Autodesk Fusion 360 part; units mm, degrees
(part 3 of 6)
  arc A637 (41.675, 81.5) -> (38.5, 78.325) centre (41.675, 78.325) ccw
  arc A638 (57.5, 78.325) -> (54.325, 81.5) centre (54.325, 78.325) ccw
  line L961 (54.325, 62.5) -> (41.675, 62.5)
  line L962 (41.675, 81.5) -> (54.325, 81.5)
  arc A639 (38.5, 65.675) -> (41.675, 62.5) centre (41.675, 65.675) ccw
  line L963 (38.5, 81.5) -> (57.5, 62.5) construction
  arc A640 (78.325, 62.5) -> (81.5, 65.675) centre (78.325, 65.675) ccw
  line L964 (62.5, 65.675) -> (62.5, 78.325)
  line L965 (81.5, 78.325) -> (81.5, 65.675)
  line L966 (81.5, 81.5) -> (62.5, 62.5) construction
  arc A641 (65.675, 81.5) -> (62.5, 78.325) centre (65.675, 78.325) ccw
  arc A642 (81.5, 78.325) -> (78.325, 81.5) centre (78.325, 78.325) ccw
  line L967 (78.325, 62.5) -> (65.675, 62.5)
  line L968 (65.675, 81.5) -> (78.325, 81.5)
  arc A643 (62.5, 65.675) -> (65.675, 62.5) centre (65.675, 65.675) ccw
  line L969 (62.5, 81.5) -> (81.5, 62.5) construction
  arc A644 (102.325, 62.5) -> (105.5, 65.675) centre (102.325, 65.675) ccw
  line L970 (86.5, 65.675) -> (86.5, 78.325)
  line L971 (105.5, 78.325) -> (105.5, 65.675)
  line L972 (105.5, 81.5) -> (86.5, 62.5) construction
  arc A645 (89.675, 81.5) -> (86.5, 78.325) centre (89.675, 78.325) ccw
  arc A646 (105.5, 78.325) -> (102.325, 81.5) centre (102.325, 78.325) ccw
  line L973 (102.325, 62.5) -> (89.675, 62.5)
  line L974 (89.675, 81.5) -> (102.325, 81.5)
  arc A647 (86.5, 65.675) -> (89.675, 62.5) centre (89.675, 65.675) ccw
  line L975 (86.5, 81.5) -> (105.5, 62.5) construction
  arc A648 (126.325, 62.5) -> (129.5, 65.675) centre (126.325, 65.675) ccw
  line L976 (110.5, 65.675) -> (110.5, 78.325)
  line L977 (129.5, 78.325) -> (129.5, 65.675)
  line L978 (129.5, 81.5) -> (110.5, 62.5) construction
  arc A649 (113.675, 81.5) -> (110.5, 78.325) centre (113.675, 78.325) ccw
  arc A650 (129.5, 78.325) -> (126.325, 81.5) centre (126.325, 78.325) ccw
  line L979 (126.325, 62.5) -> (113.675, 62.5)
  line L980 (113.675, 81.5) -> (126.325, 81.5)
  arc A651 (110.5, 65.675) -> (113.675, 62.5) centre (113.675, 65.675) ccw
  line L981 (110.5, 81.5) -> (129.5, 62.5) construction
  arc A652 (150.325, 62.5) -> (153.5, 65.675) centre (150.325, 65.675) ccw
  line L982 (134.5, 65.675) -> (134.5, 78.325)
  line L983 (153.5, 78.325) -> (153.5, 65.675)
  line L984 (153.5, 81.5) -> (134.5, 62.5) construction
  arc A653 (137.675, 81.5) -> (134.5, 78.325) centre (137.675, 78.325) ccw
  arc A654 (153.5, 78.325) -> (150.325, 81.5) centre (150.325, 78.325) ccw
  line L985 (150.325, 62.5) -> (137.675, 62.5)
  line L986 (137.675, 81.5) -> (150.325, 81.5)
  arc A655 (134.5, 65.675) -> (137.675, 62.5) centre (137.675, 65.675) ccw
  line L987 (134.5, 81.5) -> (153.5, 62.5) construction
  arc A656 (174.325, 62.5) -> (177.5, 65.675) centre (174.325, 65.675) ccw
  line L988 (158.5, 65.675) -> (158.5, 78.325)
  line L989 (177.5, 78.325) -> (177.5, 65.675)
  line L990 (177.5, 81.5) -> (158.5, 62.5) construction
  arc A657 (161.675, 81.5) -> (158.5, 78.325) centre (161.675, 78.325) ccw
  arc A658 (177.5, 78.325) -> (174.325, 81.5) centre (174.325, 78.325) ccw
  line L991 (174.325, 62.5) -> (161.675, 62.5)
  line L992 (161.675, 81.5) -> (174.325, 81.5)
  arc A659 (158.5, 65.675) -> (161.675, 62.5) centre (161.675, 65.675) ccw
  line L993 (158.5, 81.5) -> (177.5, 62.5) construction
  arc A660 (-161.675, 86.5) -> (-158.5, 89.675) centre (-161.675, 89.675) ccw
  line L994 (-177.5, 89.675) -> (-177.5, 102.325)
  line L995 (-158.5, 102.325) -> (-158.5, 89.675)
  line L996 (-158.5, 105.5) -> (-177.5, 86.5) construction
  arc A661 (-174.325, 105.5) -> (-177.5, 102.325) centre (-174.325, 102.325) ccw
  arc A662 (-158.5, 102.325) -> (-161.675, 105.5) centre (-161.675, 102.325) ccw
  line L997 (-161.675, 86.5) -> (-174.325, 86.5)
  line L998 (-174.325, 105.5) -> (-161.675, 105.5)
  arc A663 (-177.5, 89.675) -> (-174.325, 86.5) centre (-174.325, 89.675) ccw
  line L999 (-177.5, 105.5) -> (-158.5, 86.5) construction
  arc A664 (-137.675, 86.5) -> (-134.5, 89.675) centre (-137.675, 89.675) ccw
  line L1000 (-153.5, 89.675) -> (-153.5, 102.325)
  line L1001 (-134.5, 102.325) -> (-134.5, 89.675)
  line L1002 (-134.5, 105.5) -> (-153.5, 86.5) construction
  arc A665 (-150.325, 105.5) -> (-153.5, 102.325) centre (-150.325, 102.325) ccw
  arc A666 (-134.5, 102.325) -> (-137.675, 105.5) centre (-137.675, 102.325) ccw
  line L1003 (-137.675, 86.5) -> (-150.325, 86.5)
  line L1004 (-150.325, 105.5) -> (-137.675, 105.5)
  arc A667 (-153.5, 89.675) -> (-150.325, 86.5) centre (-150.325, 89.675) ccw
  line L1005 (-153.5, 105.5) -> (-134.5, 86.5) construction
  arc A668 (-113.675, 86.5) -> (-110.5, 89.675) centre (-113.675, 89.675) ccw
  line L1006 (-129.5, 89.675) -> (-129.5, 102.325)
  line L1007 (-110.5, 102.325) -> (-110.5, 89.675)
  line L1008 (-110.5, 105.5) -> (-129.5, 86.5) construction
  arc A669 (-126.325, 105.5) -> (-129.5, 102.325) centre (-126.325, 102.325) ccw
  arc A670 (-110.5, 102.325) -> (-113.675, 105.5) centre (-113.675, 102.325) ccw
  line L1009 (-113.675, 86.5) -> (-126.325, 86.5)
  line L1010 (-126.325, 105.5) -> (-113.675, 105.5)
  arc A671 (-129.5, 89.675) -> (-126.325, 86.5) centre (-126.325, 89.675) ccw
  line L1011 (-129.5, 105.5) -> (-110.5, 86.5) construction
  arc A672 (-89.675, 86.5) -> (-86.5, 89.675) centre (-89.675, 89.675) ccw
  line L1012 (-105.5, 89.675) -> (-105.5, 102.325)
  line L1013 (-86.5, 102.325) -> (-86.5, 89.675)
  line L1014 (-86.5, 105.5) -> (-105.5, 86.5) construction
  arc A673 (-102.325, 105.5) -> (-105.5, 102.325) centre (-102.325, 102.325) ccw
  arc A674 (-86.5, 102.325) -> (-89.675, 105.5) centre (-89.675, 102.325) ccw
  line L1015 (-89.675, 86.5) -> (-102.325, 86.5)
  line L1016 (-102.325, 105.5) -> (-89.675, 105.5)
  arc A675 (-105.5, 89.675) -> (-102.325, 86.5) centre (-102.325, 89.675) ccw
  line L1017 (-105.5, 105.5) -> (-86.5, 86.5) construction
  arc A676 (-65.675, 86.5) -> (-62.5, 89.675) centre (-65.675, 89.675) ccw
  line L1018 (-81.5, 89.675) -> (-81.5, 102.325)
  line L1019 (-62.5, 102.325) -> (-62.5, 89.675)
  line L1020 (-62.5, 105.5) -> (-81.5, 86.5) construction
  arc A677 (-78.325, 105.5) -> (-81.5, 102.325) centre (-78.325, 102.325) ccw
  arc A678 (-62.5, 102.325) -> (-65.675, 105.5) centre (-65.675, 102.325) ccw
  line L1021 (-65.675, 86.5) -> (-78.325, 86.5)
  line L1022 (-78.325, 105.5) -> (-65.675, 105.5)
  arc A679 (-81.5, 89.675) -> (-78.325, 86.5) centre (-78.325, 89.675) ccw
  line L1023 (-81.5, 105.5) -> (-62.5, 86.5) construction
  arc A680 (-41.675, 86.5) -> (-38.5, 89.675) centre (-41.675, 89.675) ccw
  line L1024 (-57.5, 89.675) -> (-57.5, 102.325)
  line L1025 (-38.5, 102.325) -> (-38.5, 89.675)
  line L1026 (-38.5, 105.5) -> (-57.5, 86.5) construction
  arc A681 (-54.325, 105.5) -> (-57.5, 102.325) centre (-54.325, 102.325) ccw
  arc A682 (-38.5, 102.325) -> (-41.675, 105.5) centre (-41.675, 102.325) ccw
  line L1027 (-41.675, 86.5) -> (-54.325, 86.5)
  line L1028 (-54.325, 105.5) -> (-41.675, 105.5)
  arc A683 (-57.5, 89.675) -> (-54.325, 86.5) centre (-54.325, 89.675) ccw
  line L1029 (-57.5, 105.5) -> (-38.5, 86.5) construction
  arc A684 (-17.675, 86.5) -> (-14.5, 89.675) centre (-17.675, 89.675) ccw
  line L1030 (-33.5, 89.675) -> (-33.5, 102.325)
  line L1031 (-14.5, 102.325) -> (-14.5, 89.675)
  line L1032 (-14.5, 105.5) -> (-33.5, 86.5) construction
  arc A685 (-30.325, 105.5) -> (-33.5, 102.325) centre (-30.325, 102.325) ccw
  arc A686 (-14.5, 102.325) -> (-17.675, 105.5) centre (-17.675, 102.325) ccw
  line L1033 (-17.675, 86.5) -> (-30.325, 86.5)
  line L1034 (-30.325, 105.5) -> (-17.675, 105.5)
  arc A687 (-33.5, 89.675) -> (-30.325, 86.5) centre (-30.325, 89.675) ccw
  line L1035 (-33.5, 105.5) -> (-14.5, 86.5) construction
  arc A688 (6.325, 86.5) -> (9.5, 89.675) centre (6.325, 89.675) ccw
  line L1036 (-9.5, 89.675) -> (-9.5, 102.325)
  line L1037 (9.5, 102.325) -> (9.5, 89.675)
  line L1038 (9.5, 105.5) -> (-9.5, 86.5) construction
  arc A689 (-6.325, 105.5) -> (-9.5, 102.325) centre (-6.325, 102.325) ccw
  arc A690 (9.5, 102.325) -> (6.325, 105.5) centre (6.325, 102.325) ccw
  line L1039 (6.325, 86.5) -> (-6.325, 86.5)
  line L1040 (-6.325, 105.5) -> (6.325, 105.5)
  arc A691 (-9.5, 89.675) -> (-6.325, 86.5) centre (-6.325, 89.675) ccw
  line L1041 (-9.5, 105.5) -> (9.5, 86.5) construction
  arc A692 (30.325, 86.5) -> (33.5, 89.675) centre (30.325, 89.675) ccw
  line L1042 (14.5, 89.675) -> (14.5, 102.325)
  line L1043 (33.5, 102.325) -> (33.5, 89.675)
  line L1044 (33.5, 105.5) -> (14.5, 86.5) construction
  arc A693 (17.675, 105.5) -> (14.5, 102.325) centre (17.675, 102.325) ccw
  arc A694 (33.5, 102.325) -> (30.325, 105.5) centre (30.325, 102.325) ccw
  line L1045 (30.325, 86.5) -> (17.675, 86.5)
  line L1046 (17.675, 105.5) -> (30.325, 105.5)
  arc A695 (14.5, 89.675) -> (17.675, 86.5) centre (17.675, 89.675) ccw
  line L1047 (14.5, 105.5) -> (33.5, 86.5) construction
  arc A696 (54.325, 86.5) -> (57.5, 89.675) centre (54.325, 89.675) ccw
  line L1048 (38.5, 89.675) -> (38.5, 102.325)
  line L1049 (57.5, 102.325) -> (57.5, 89.675)
  line L1050 (57.5, 105.5) -> (38.5, 86.5) construction
  arc A697 (41.675, 105.5) -> (38.5, 102.325) centre (41.675, 102.325) ccw
  arc A698 (57.5, 102.325) -> (54.325, 105.5) centre (54.325, 102.325) ccw
  line L1051 (54.325, 86.5) -> (41.675, 86.5)
  line L1052 (41.675, 105.5) -> (54.325, 105.5)
  arc A699 (38.5, 89.675) -> (41.675, 86.5) centre (41.675, 89.675) ccw
  line L1053 (38.5, 105.5) -> (57.5, 86.5) construction
  arc A700 (78.325, 86.5) -> (81.5, 89.675) centre (78.325, 89.675) ccw
  line L1054 (62.5, 89.675) -> (62.5, 102.325)
  line L1055 (81.5, 102.325) -> (81.5, 89.675)
  line L1056 (81.5, 105.5) -> (62.5, 86.5) construction
  arc A701 (65.675, 105.5) -> (62.5, 102.325) centre (65.675, 102.325) ccw
  arc A702 (81.5, 102.325) -> (78.325, 105.5) centre (78.325, 102.325) ccw
  line L1057 (78.325, 86.5) -> (65.675, 86.5)
  line L1058 (65.675, 105.5) -> (78.325, 105.5)
  arc A703 (62.5, 89.675) -> (65.675, 86.5) centre (65.675, 89.675) ccw
  line L1059 (62.5, 105.5) -> (81.5, 86.5) construction
  arc A704 (102.325, 86.5) -> (105.5, 89.675) centre (102.325, 89.675) ccw
  line L1060 (86.5, 89.675) -> (86.5, 102.325)
  line L1061 (105.5, 102.325) -> (105.5, 89.675)
  line L1062 (105.5, 105.5) -> (86.5, 86.5) construction
  arc A705 (89.675, 105.5) -> (86.5, 102.325) centre (89.675, 102.325) ccw
  arc A706 (105.5, 102.325) -> (102.325, 105.5) centre (102.325, 102.325) ccw
  line L1063 (102.325, 86.5) -> (89.675, 86.5)
  line L1064 (89.675, 105.5) -> (102.325, 105.5)
  arc A707 (86.5, 89.675) -> (89.675, 86.5) centre (89.675, 89.675) ccw
  line L1065 (86.5, 105.5) -> (105.5, 86.5) construction
  arc A708 (126.325, 86.5) -> (129.5, 89.675) centre (126.325, 89.675) ccw
  line L1066 (110.5, 89.675) -> (110.5, 102.325)
  line L1067 (129.5, 102.325) -> (129.5, 89.675)
  line L1068 (129.5, 105.5) -> (110.5, 86.5) construction
  arc A709 (113.675, 105.5) -> (110.5, 102.325) centre (113.675, 102.325) ccw
  arc A710 (129.5, 102.325) -> (126.325, 105.5) centre (126.325, 102.325) ccw
  line L1069 (126.325, 86.5) -> (113.675, 86.5)
  line L1070 (113.675, 105.5) -> (126.325, 105.5)
  arc A711 (110.5, 89.675) -> (113.675, 86.5) centre (113.675, 89.675) ccw
  line L1071 (110.5, 105.5) -> (129.5, 86.5) construction
  arc A712 (150.325, 86.5) -> (153.5, 89.675) centre (150.325, 89.675) ccw
  line L1072 (134.5, 89.675) -> (134.5, 102.325)
  line L1073 (153.5, 102.325) -> (153.5, 89.675)
  line L1074 (153.5, 105.5) -> (134.5, 86.5) construction
  arc A713 (137.675, 105.5) -> (134.5, 102.325) centre (137.675, 102.325) ccw
  arc A714 (153.5, 102.325) -> (150.325, 105.5) centre (150.325, 102.325) ccw
  line L1075 (150.325, 86.5) -> (137.675, 86.5)
  line L1076 (137.675, 105.5) -> (150.325, 105.5)
  arc A715 (134.5, 89.675) -> (137.675, 86.5) centre (137.675, 89.675) ccw
  line L1077 (134.5, 105.5) -> (153.5, 86.5) construction
  arc A716 (174.325, 86.5) -> (177.5, 89.675) centre (174.325, 89.675) ccw
  line L1078 (158.5, 89.675) -> (158.5, 102.325)
  line L1079 (177.5, 102.325) -> (177.5, 89.675)
  line L1080 (177.5, 105.5) -> (158.5, 86.5) construction
  arc A717 (161.675, 105.5) -> (158.5, 102.325) centre (161.675, 102.325) ccw
  arc A718 (177.5, 102.325) -> (174.325, 105.5) centre (174.325, 102.325) ccw
  line L1081 (174.325, 86.5) -> (161.675, 86.5)
  line L1082 (161.675, 105.5) -> (174.325, 105.5)
  arc A719 (158.5, 89.675) -> (161.675, 86.5) centre (161.675, 89.675) ccw
  line L1083 (158.5, 105.5) -> (177.5, 86.5) construction
  arc A720 (-161.675, 110.5) -> (-158.5, 113.675) centre (-161.675, 113.675) ccw
  line L1084 (-177.5, 113.675) -> (-177.5, 126.325)
  line L1085 (-158.5, 126.325) -> (-158.5, 113.675)
  line L1086 (-158.5, 129.5) -> (-177.5, 110.5) construction
  arc A721 (-174.325, 129.5) -> (-177.5, 126.325) centre (-174.325, 126.325) ccw
  arc A722 (-158.5, 126.325) -> (-161.675, 129.5) centre (-161.675, 126.325) ccw
  line L1087 (-161.675, 110.5) -> (-174.325, 110.5)
  line L1088 (-174.325, 129.5) -> (-161.675, 129.5)
  arc A723 (-177.5, 113.675) -> (-174.325, 110.5) centre (-174.325, 113.675) ccw
  line L1089 (-177.5, 129.5) -> (-158.5, 110.5) construction
  arc A724 (-137.675, 110.5) -> (-134.5, 113.675) centre (-137.675, 113.675) ccw
  line L1090 (-153.5, 113.675) -> (-153.5, 126.325)
  line L1091 (-134.5, 126.325) -> (-134.5, 113.675)
  line L1092 (-134.5, 129.5) -> (-153.5, 110.5) construction
  arc A725 (-150.325, 129.5) -> (-153.5, 126.325) centre (-150.325, 126.325) ccw
  arc A726 (-134.5, 126.325) -> (-137.675, 129.5) centre (-137.675, 126.325) ccw
  line L1093 (-137.675, 110.5) -> (-150.325, 110.5)
  line L1094 (-150.325, 129.5) -> (-137.675, 129.5)
  arc A727 (-153.5, 113.675) -> (-150.325, 110.5) centre (-150.325, 113.675) ccw
  line L1095 (-153.5, 129.5) -> (-134.5, 110.5) construction
  arc A728 (-113.675, 110.5) -> (-110.5, 113.675) centre (-113.675, 113.675) ccw
  line L1096 (-129.5, 113.675) -> (-129.5, 126.325)
  line L1097 (-110.5, 126.325) -> (-110.5, 113.675)
  line L1098 (-110.5, 129.5) -> (-129.5, 110.5) construction
  arc A729 (-126.325, 129.5) -> (-129.5, 126.325) centre (-126.325, 126.325) ccw
  arc A730 (-110.5, 126.325) -> (-113.675, 129.5) centre (-113.675, 126.325) ccw
  line L1099 (-113.675, 110.5) -> (-126.325, 110.5)
  line L1100 (-126.325, 129.5) -> (-113.675, 129.5)
  arc A731 (-129.5, 113.675) -> (-126.325, 110.5) centre (-126.325, 113.675) ccw
  line L1101 (-129.5, 129.5) -> (-110.5, 110.5) construction
  arc A732 (-89.675, 110.5) -> (-86.5, 113.675) centre (-89.675, 113.675) ccw
  line L1102 (-105.5, 113.675) -> (-105.5, 126.325)
  line L1103 (-86.5, 126.325) -> (-86.5, 113.675)
  line L1104 (-86.5, 129.5) -> (-105.5, 110.5) construction
  arc A733 (-102.325, 129.5) -> (-105.5, 126.325) centre (-102.325, 126.325) ccw
  arc A734 (-86.5, 126.325) -> (-89.675, 129.5) centre (-89.675, 126.325) ccw
  line L1105 (-89.675, 110.5) -> (-102.325, 110.5)
  line L1106 (-102.325, 129.5) -> (-89.675, 129.5)
  arc A735 (-105.5, 113.675) -> (-102.325, 110.5) centre (-102.325, 113.675) ccw
  line L1107 (-105.5, 129.5) -> (-86.5, 110.5) construction
  arc A736 (-65.675, 110.5) -> (-62.5, 113.675) centre (-65.675, 113.675) ccw
  line L1108 (-81.5, 113.675) -> (-81.5, 126.325)
  line L1109 (-62.5, 126.325) -> (-62.5, 113.675)
  line L1110 (-62.5, 129.5) -> (-81.5, 110.5) construction
  arc A737 (-78.325, 129.5) -> (-81.5, 126.325) centre (-78.325, 126.325) ccw
  arc A738 (-62.5, 126.325) -> (-65.675, 129.5) centre (-65.675, 126.325) ccw
  line L1111 (-65.675, 110.5) -> (-78.325, 110.5)
  line L1112 (-78.325, 129.5) -> (-65.675, 129.5)
  arc A739 (-81.5, 113.675) -> (-78.325, 110.5) centre (-78.325, 113.675) ccw
  line L1113 (-81.5, 129.5) -> (-62.5, 110.5) construction
  arc A740 (-41.675, 110.5) -> (-38.5, 113.675) centre (-41.675, 113.675) ccw
  line L1114 (-57.5, 113.675) -> (-57.5, 126.325)
  line L1115 (-38.5, 126.325) -> (-38.5, 113.675)
  line L1116 (-38.5, 129.5) -> (-57.5, 110.5) construction
  arc A741 (-54.325, 129.5) -> (-57.5, 126.325) centre (-54.325, 126.325) ccw
  arc A742 (-38.5, 126.325) -> (-41.675, 129.5) centre (-41.675, 126.325) ccw
  line L1117 (-41.675, 110.5) -> (-54.325, 110.5)
  line L1118 (-54.325, 129.5) -> (-41.675, 129.5)
  arc A743 (-57.5, 113.675) -> (-54.325, 110.5) centre (-54.325, 113.675) ccw
  line L1119 (-57.5, 129.5) -> (-38.5, 110.5) construction
  arc A744 (-17.675, 110.5) -> (-14.5, 113.675) centre (-17.675, 113.675) ccw
  line L1120 (-33.5, 113.675) -> (-33.5, 126.325)
  line L1121 (-14.5, 126.325) -> (-14.5, 113.675)
  line L1122 (-14.5, 129.5) -> (-33.5, 110.5) construction
  arc A745 (-30.325, 129.5) -> (-33.5, 126.325) centre (-30.325, 126.325) ccw
  arc A746 (-14.5, 126.325) -> (-17.675, 129.5) centre (-17.675, 126.325) ccw
  line L1123 (-17.675, 110.5) -> (-30.325, 110.5)
  line L1124 (-30.325, 129.5) -> (-17.675, 129.5)
  arc A747 (-33.5, 113.675) -> (-30.325, 110.5) centre (-30.325, 113.675) ccw
  line L1125 (-33.5, 129.5) -> (-14.5, 110.5) construction
  arc A748 (6.325, 110.5) -> (9.5, 113.675) centre (6.325, 113.675) ccw
  line L1126 (-9.5, 113.675) -> (-9.5, 126.325)
  line L1127 (9.5, 126.325) -> (9.5, 113.675)
  line L1128 (9.5, 129.5) -> (-9.5, 110.5) construction
  arc A749 (-6.325, 129.5) -> (-9.5, 126.325) centre (-6.325, 126.325) ccw
  arc A750 (9.5, 126.325) -> (6.325, 129.5) centre (6.325, 126.325) ccw
  line L1129 (6.325, 110.5) -> (-6.325, 110.5)
  line L1130 (-6.325, 129.5) -> (6.325, 129.5)
  arc A751 (-9.5, 113.675) -> (-6.325, 110.5) centre (-6.325, 113.675) ccw
  line L1131 (-9.5, 129.5) -> (9.5, 110.5) construction
  arc A752 (30.325, 110.5) -> (33.5, 113.675) centre (30.325, 113.675) ccw
  line L1132 (14.5, 113.675) -> (14.5, 126.325)
  line L1133 (33.5, 126.325) -> (33.5, 113.675)
  line L1134 (33.5, 129.5) -> (14.5, 110.5) construction
  arc A753 (17.675, 129.5) -> (14.5, 126.325) centre (17.675, 126.325) ccw
  arc A754 (33.5, 126.325) -> (30.325, 129.5) centre (30.325, 126.325) ccw
  line L1135 (30.325, 110.5) -> (17.675, 110.5)
  line L1136 (17.675, 129.5) -> (30.325, 129.5)
  arc A755 (14.5, 113.675) -> (17.675, 110.5) centre (17.675, 113.675) ccw
  line L1137 (14.5, 129.5) -> (33.5, 110.5) construction
  arc A756 (54.325, 110.5) -> (57.5, 113.675) centre (54.325, 113.675) ccw
  line L1138 (38.5, 113.675) -> (38.5, 126.325)
  line L1139 (57.5, 126.325) -> (57.5, 113.675)
  line L1140 (57.5, 129.5) -> (38.5, 110.5) construction
  arc A757 (41.675, 129.5) -> (38.5, 126.325) centre (41.675, 126.325) ccw
  arc A758 (57.5, 126.325) -> (54.325, 129.5) centre (54.325, 126.325) ccw
  line L1141 (54.325, 110.5) -> (41.675, 110.5)
  line L1142 (41.675, 129.5) -> (54.325, 129.5)
  arc A759 (38.5, 113.675) -> (41.675, 110.5) centre (41.675, 113.675) ccw
  line L1143 (38.5, 129.5) -> (57.5, 110.5) construction
  arc A760 (78.325, 110.5) -> (81.5, 113.675) centre (78.325, 113.675) ccw
  line L1144 (62.5, 113.675) -> (62.5, 126.325)
  line L1145 (81.5, 126.325) -> (81.5, 113.675)
  line L1146 (81.5, 129.5) -> (62.5, 110.5) construction
  arc A761 (65.675, 129.5) -> (62.5, 126.325) centre (65.675, 126.325) ccw
  arc A762 (81.5, 126.325) -> (78.325, 129.5) centre (78.325, 126.325) ccw
  line L1147 (78.325, 110.5) -> (65.675, 110.5)
  line L1148 (65.675, 129.5) -> (78.325, 129.5)
  arc A763 (62.5, 113.675) -> (65.675, 110.5) centre (65.675, 113.675) ccw
  line L1149 (62.5, 129.5) -> (81.5, 110.5) construction
  arc A764 (102.325, 110.5) -> (105.5, 113.675) centre (102.325, 113.675) ccw
  line L1150 (86.5, 113.675) -> (86.5, 126.325)
  line L1151 (105.5, 126.325) -> (105.5, 113.675)
  line L1152 (105.5, 129.5) -> (86.5, 110.5) construction
  arc A765 (89.675, 129.5) -> (86.5, 126.325) centre (89.675, 126.325) ccw
  arc A766 (105.5, 126.325) -> (102.325, 129.5) centre (102.325, 126.325) ccw
  line L1153 (102.325, 110.5) -> (89.675, 110.5)
  line L1154 (89.675, 129.5) -> (102.325, 129.5)
  arc A767 (86.5, 113.675) -> (89.675, 110.5) centre (89.675, 113.675) ccw
  line L1155 (86.5, 129.5) -> (105.5, 110.5) construction
  arc A768 (126.325, 110.5) -> (129.5, 113.675) centre (126.325, 113.675) ccw
  line L1156 (110.5, 113.675) -> (110.5, 126.325)
  line L1157 (129.5, 126.325) -> (129.5, 113.675)
  line L1158 (129.5, 129.5) -> (110.5, 110.5) construction
  arc A769 (113.675, 129.5) -> (110.5, 126.325) centre (113.675, 126.325) ccw
  arc A770 (129.5, 126.325) -> (126.325, 129.5) centre (126.325, 126.325) ccw
  line L1159 (126.325, 110.5) -> (113.675, 110.5)
  line L1160 (113.675, 129.5) -> (126.325, 129.5)
  arc A771 (110.5, 113.675) -> (113.675, 110.5) centre (113.675, 113.675) ccw
  line L1161 (110.5, 129.5) -> (129.5, 110.5) construction
  arc A772 (150.325, 110.5) -> (153.5, 113.675) centre (150.325, 113.675) ccw
  line L1162 (134.5, 113.675) -> (134.5, 126.325)
  line L1163 (153.5, 126.325) -> (153.5, 113.675)
  line L1164 (153.5, 129.5) -> (134.5, 110.5) construction
  arc A773 (137.675, 129.5) -> (134.5, 126.325) centre (137.675, 126.325) ccw
  arc A774 (153.5, 126.325) -> (150.325, 129.5) centre (150.325, 126.325) ccw
  line L1165 (150.325, 110.5) -> (137.675, 110.5)
  line L1166 (137.675, 129.5) -> (150.325, 129.5)
  arc A775 (134.5, 113.675) -> (137.675, 110.5) centre (137.675, 113.675) ccw
  line L1167 (134.5, 129.5) -> (153.5, 110.5) construction
  arc A776 (174.325, 110.5) -> (177.5, 113.675) centre (174.325, 113.675) ccw
  line L1168 (158.5, 113.675) -> (158.5, 126.325)
  line L1169 (177.5, 126.325) -> (177.5, 113.675)
  line L1170 (177.5, 129.5) -> (158.5, 110.5) construction
  arc A777 (161.675, 129.5) -> (158.5, 126.325) centre (161.675, 126.325) ccw
  arc A778 (177.5, 126.325) -> (174.325, 129.5) centre (174.325, 126.325) ccw
  line L1171 (174.325, 110.5) -> (161.675, 110.5)
  line L1172 (161.675, 129.5) -> (174.325, 129.5)
  arc A779 (158.5, 113.675) -> (161.675, 110.5) centre (161.675, 113.675) ccw
  line L1173 (158.5, 129.5) -> (177.5, 110.5) construction
  arc A780 (-161.675, 134.5) -> (-158.5, 137.675) centre (-161.675, 137.675) ccw
  line L1174 (-177.5, 137.675) -> (-177.5, 150.325)
  line L1175 (-158.5, 150.325) -> (-158.5, 137.675)
  line L1176 (-158.5, 153.5) -> (-177.5, 134.5) construction
  arc A781 (-174.325, 153.5) -> (-177.5, 150.325) centre (-174.325, 150.325) ccw
  arc A782 (-158.5, 150.325) -> (-161.675, 153.5) centre (-161.675, 150.325) ccw
  line L1177 (-161.675, 134.5) -> (-174.325, 134.5)
  line L1178 (-174.325, 153.5) -> (-161.675, 153.5)
  arc A783 (-177.5, 137.675) -> (-174.325, 134.5) centre (-174.325, 137.675) ccw
  line L1179 (-177.5, 153.5) -> (-158.5, 134.5) construction
  arc A784 (-137.675, 134.5) -> (-134.5, 137.675) centre (-137.675, 137.675) ccw
  line L1180 (-153.5, 137.675) -> (-153.5, 150.325)
  line L1181 (-134.5, 150.325) -> (-134.5, 137.675)
  line L1182 (-134.5, 153.5) -> (-153.5, 134.5) construction
  arc A785 (-150.325, 153.5) -> (-153.5, 150.325) centre (-150.325, 150.325) ccw
  arc A786 (-134.5, 150.325) -> (-137.675, 153.5) centre (-137.675, 150.325) ccw
  line L1183 (-137.675, 134.5) -> (-150.325, 134.5)
  line L1184 (-150.325, 153.5) -> (-137.675, 153.5)
  arc A787 (-153.5, 137.675) -> (-150.325, 134.5) centre (-150.325, 137.675) ccw
  line L1185 (-153.5, 153.5) -> (-134.5, 134.5) construction
  arc A788 (-113.675, 134.5) -> (-110.5, 137.675) centre (-113.675, 137.675) ccw
  line L1186 (-129.5, 137.675) -> (-129.5, 150.325)
  line L1187 (-110.5, 150.325) -> (-110.5, 137.675)
  line L1188 (-110.5, 153.5) -> (-129.5, 134.5) construction
  arc A789 (-126.325, 153.5) -> (-129.5, 150.325) centre (-126.325, 150.325) ccw
  arc A790 (-110.5, 150.325) -> (-113.675, 153.5) centre (-113.675, 150.325) ccw
  line L1189 (-113.675, 134.5) -> (-126.325, 134.5)
  line L1190 (-126.325, 153.5) -> (-113.675, 153.5)
  arc A791 (-129.5, 137.675) -> (-126.325, 134.5) centre (-126.325, 137.675) ccw
  line L1191 (-129.5, 153.5) -> (-110.5, 134.5) construction
  arc A792 (-89.675, 134.5) -> (-86.5, 137.675) centre (-89.675, 137.675) ccw
  line L1192 (-105.5, 137.675) -> (-105.5, 150.325)
  line L1193 (-86.5, 150.325) -> (-86.5, 137.675)
  line L1194 (-86.5, 153.5) -> (-105.5, 134.5) construction
  arc A793 (-102.325, 153.5) -> (-105.5, 150.325) centre (-102.325, 150.325) ccw
  arc A794 (-86.5, 150.325) -> (-89.675, 153.5) centre (-89.675, 150.325) ccw
  line L1195 (-89.675, 134.5) -> (-102.325, 134.5)
  line L1196 (-102.325, 153.5) -> (-89.675, 153.5)
  arc A795 (-105.5, 137.675) -> (-102.325, 134.5) centre (-102.325, 137.675) ccw
  line L1197 (-105.5, 153.5) -> (-86.5, 134.5) construction
  arc A796 (-65.675, 134.5) -> (-62.5, 137.675) centre (-65.675, 137.675) ccw
  line L1198 (-81.5, 137.675) -> (-81.5, 150.325)
  line L1199 (-62.5, 150.325) -> (-62.5, 137.675)
  line L1200 (-62.5, 153.5) -> (-81.5, 134.5) construction
  arc A797 (-78.325, 153.5) -> (-81.5, 150.325) centre (-78.325, 150.325) ccw
  arc A798 (-62.5, 150.325) -> (-65.675, 153.5) centre (-65.675, 150.325) ccw
  line L1201 (-65.675, 134.5) -> (-78.325, 134.5)
  line L1202 (-78.325, 153.5) -> (-65.675, 153.5)
  arc A799 (-81.5, 137.675) -> (-78.325, 134.5) centre (-78.325, 137.675) ccw
  line L1203 (-81.5, 153.5) -> (-62.5, 134.5) construction
  arc A800 (-41.675, 134.5) -> (-38.5, 137.675) centre (-41.675, 137.675) ccw
  line L1204 (-57.5, 137.675) -> (-57.5, 150.325)
  line L1205 (-38.5, 150.325) -> (-38.5, 137.675)
  line L1206 (-38.5, 153.5) -> (-57.5, 134.5) construction
  arc A801 (-54.325, 153.5) -> (-57.5, 150.325) centre (-54.325, 150.325) ccw
  arc A802 (-38.5, 150.325) -> (-41.675, 153.5) centre (-41.675, 150.325) ccw
  line L1207 (-41.675, 134.5) -> (-54.325, 134.5)
  line L1208 (-54.325, 153.5) -> (-41.675, 153.5)
  arc A803 (-57.5, 137.675) -> (-54.325, 134.5) centre (-54.325, 137.675) ccw
  line L1209 (-57.5, 153.5) -> (-38.5, 134.5) construction
  arc A804 (-17.675, 134.5) -> (-14.5, 137.675) centre (-17.675, 137.675) ccw
  line L1210 (-33.5, 137.675) -> (-33.5, 150.325)
  line L1211 (-14.5, 150.325) -> (-14.5, 137.675)
  line L1212 (-14.5, 153.5) -> (-33.5, 134.5) construction
  arc A805 (-30.325, 153.5) -> (-33.5, 150.325) centre (-30.325, 150.325) ccw
  arc A806 (-14.5, 150.325) -> (-17.675, 153.5) centre (-17.675, 150.325) ccw
  line L1213 (-17.675, 134.5) -> (-30.325, 134.5)
  line L1214 (-30.325, 153.5) -> (-17.675, 153.5)
  arc A807 (-33.5, 137.675) -> (-30.325, 134.5) centre (-30.325, 137.675) ccw
  line L1215 (-33.5, 153.5) -> (-14.5, 134.5) construction
  arc A808 (6.325, 134.5) -> (9.5, 137.675) centre (6.325, 137.675) ccw
  line L1216 (-9.5, 137.675) -> (-9.5, 150.325)
  line L1217 (9.5, 150.325) -> (9.5, 137.675)
  line L1218 (9.5, 153.5) -> (-9.5, 134.5) construction
  arc A809 (-6.325, 153.5) -> (-9.5, 150.325) centre (-6.325, 150.325) ccw
  arc A810 (9.5, 150.325) -> (6.325, 153.5) centre (6.325, 150.325) ccw
  line L1219 (6.325, 134.5) -> (-6.325, 134.5)
  line L1220 (-6.325, 153.5) -> (6.325, 153.5)
  arc A811 (-9.5, 137.675) -> (-6.325, 134.5) centre (-6.325, 137.675) ccw
  line L1221 (-9.5, 153.5) -> (9.5, 134.5) construction
  arc A812 (30.325, 134.5) -> (33.5, 137.675) centre (30.325, 137.675) ccw
  line L1222 (14.5, 137.675) -> (14.5, 150.325)
  line L1223 (33.5, 150.325) -> (33.5, 137.675)
  line L1224 (33.5, 153.5) -> (14.5, 134.5) construction
  arc A813 (17.675, 153.5) -> (14.5, 150.325) centre (17.675, 150.325) ccw
  arc A814 (33.5, 150.325) -> (30.325, 153.5) centre (30.325, 150.325) ccw
  line L1225 (30.325, 134.5) -> (17.675, 134.5)
  line L1226 (17.675, 153.5) -> (30.325, 153.5)
  arc A815 (14.5, 137.675) -> (17.675, 134.5) centre (17.675, 137.675) ccw
  line L1227 (14.5, 153.5) -> (33.5, 134.5) construction
  arc A816 (54.325, 134.5) -> (57.5, 137.675) centre (54.325, 137.675) ccw
  line L1228 (38.5, 137.675) -> (38.5, 150.325)
  line L1229 (57.5, 150.325) -> (57.5, 137.675)
  line L1230 (57.5, 153.5) -> (38.5, 134.5) construction
  arc A817 (41.675, 153.5) -> (38.5, 150.325) centre (41.675, 150.325) ccw
  arc A818 (57.5, 150.325) -> (54.325, 153.5) centre (54.325, 150.325) ccw
  line L1231 (54.325, 134.5) -> (41.675, 134.5)
  line L1232 (41.675, 153.5) -> (54.325, 153.5)
  arc A819 (38.5, 137.675) -> (41.675, 134.5) centre (41.675, 137.675) ccw
  line L1233 (38.5, 153.5) -> (57.5, 134.5) construction
  arc A820 (78.325, 134.5) -> (81.5, 137.675) centre (78.325, 137.675) ccw
  line L1234 (62.5, 137.675) -> (62.5, 150.325)
  line L1235 (81.5, 150.325) -> (81.5, 137.675)
  line L1236 (81.5, 153.5) -> (62.5, 134.5) construction
  arc A821 (65.675, 153.5) -> (62.5, 150.325) centre (65.675, 150.325) ccw
  arc A822 (81.5, 150.325) -> (78.325, 153.5) centre (78.325, 150.325) ccw
  line L1237 (78.325, 134.5) -> (65.675, 134.5)
  line L1238 (65.675, 153.5) -> (78.325, 153.5)
  arc A823 (62.5, 137.675) -> (65.675, 134.5) centre (65.675, 137.675) ccw
  line L1239 (62.5, 153.5) -> (81.5, 134.5) construction
  arc A824 (102.325, 134.5) -> (105.5, 137.675) centre (102.325, 137.675) ccw
  line L1240 (86.5, 137.675) -> (86.5, 150.325)
  line L1241 (105.5, 150.325) -> (105.5, 137.675)
  line L1242 (105.5, 153.5) -> (86.5, 134.5) construction
  arc A825 (89.675, 153.5) -> (86.5, 150.325) centre (89.675, 150.325) ccw
  arc A826 (105.5, 150.325) -> (102.325, 153.5) centre (102.325, 150.325) ccw
  line L1243 (102.325, 134.5) -> (89.675, 134.5)
  line L1244 (89.675, 153.5) -> (102.325, 153.5)
  arc A827 (86.5, 137.675) -> (89.675, 134.5) centre (89.675, 137.675) ccw
  line L1245 (86.5, 153.5) -> (105.5, 134.5) construction
  arc A828 (126.325, 134.5) -> (129.5, 137.675) centre (126.325, 137.675) ccw
  line L1246 (110.5, 137.675) -> (110.5, 150.325)
  line L1247 (129.5, 150.325) -> (129.5, 137.675)
  line L1248 (129.5, 153.5) -> (110.5, 134.5) construction
  arc A829 (113.675, 153.5) -> (110.5, 150.325) centre (113.675, 150.325) ccw
  arc A830 (129.5, 150.325) -> (126.325, 153.5) centre (126.325, 150.325) ccw
  line L1249 (126.325, 134.5) -> (113.675, 134.5)
  line L1250 (113.675, 153.5) -> (126.325, 153.5)
  arc A831 (110.5, 137.675) -> (113.675, 134.5) centre (113.675, 137.675) ccw
  line L1251 (110.5, 153.5) -> (129.5, 134.5) construction
  arc A832 (150.325, 134.5) -> (153.5, 137.675) centre (150.325, 137.675) ccw
  line L1252 (134.5, 137.675) -> (134.5, 150.325)
  line L1253 (153.5, 150.325) -> (153.5, 137.675)
  line L1254 (153.5, 153.5) -> (134.5, 134.5) construction
  arc A833 (137.675, 153.5) -> (134.5, 150.325) centre (137.675, 150.325) ccw
  arc A834 (153.5, 150.325) -> (150.325, 153.5) centre (150.325, 150.325) ccw
  line L1255 (150.325, 134.5) -> (137.675, 134.5)
  line L1256 (137.675, 153.5) -> (150.325, 153.5)
  arc A835 (134.5, 137.675) -> (137.675, 134.5) centre (137.675, 137.675) ccw
  line L1257 (134.5, 153.5) -> (153.5, 134.5) construction
  arc A836 (174.325, 134.5) -> (177.5, 137.675) centre (174.325, 137.675) ccw
  line L1258 (158.5, 137.675) -> (158.5, 150.325)
  line L1259 (177.5, 150.325) -> (177.5, 137.675)
  line L1260 (177.5, 153.5) -> (158.5, 134.5) construction
  arc A837 (161.675, 153.5) -> (158.5, 150.325) centre (161.675, 150.325) ccw
  arc A838 (177.5, 150.325) -> (174.325, 153.5) centre (174.325, 150.325) ccw
  line L1261 (174.325, 134.5) -> (161.675, 134.5)
  line L1262 (161.675, 153.5) -> (174.325, 153.5)
  arc A839 (158.5, 137.675) -> (161.675, 134.5) centre (161.675, 137.675) ccw
  line L1263 (158.5, 153.5) -> (177.5, 134.5) construction
  arc A840 (-161.675, 158.5) -> (-158.5, 161.675) centre (-161.675, 161.675) ccw
  line L1264 (-177.5, 161.675) -> (-177.5, 174.325)
  line L1265 (-158.5, 174.325) -> (-158.5, 161.675)
  line L1266 (-158.5, 177.5) -> (-177.5, 158.5) construction
  arc A841 (-174.325, 177.5) -> (-177.5, 174.325) centre (-174.325, 174.325) ccw
  arc A842 (-158.5, 174.325) -> (-161.675, 177.5) centre (-161.675, 174.325) ccw
  line L1267 (-161.675, 158.5) -> (-174.325, 158.5)
  line L1268 (-174.325, 177.5) -> (-161.675, 177.5)
  arc A843 (-177.5, 161.675) -> (-174.325, 158.5) centre (-174.325, 161.675) ccw
  line L1269 (-177.5, 177.5) -> (-158.5, 158.5) construction
  arc A844 (-137.675, 158.5) -> (-134.5, 161.675) centre (-137.675, 161.675) ccw
  line L1270 (-153.5, 161.675) -> (-153.5, 174.325)
  line L1271 (-134.5, 174.325) -> (-134.5, 161.675)
  line L1272 (-134.5, 177.5) -> (-153.5, 158.5) construction
  arc A845 (-150.325, 177.5) -> (-153.5, 174.325) centre (-150.325, 174.325) ccw
  arc A846 (-134.5, 174.325) -> (-137.675, 177.5) centre (-137.675, 174.325) ccw
  line L1273 (-137.675, 158.5) -> (-150.325, 158.5)
  line L1274 (-150.325, 177.5) -> (-137.675, 177.5)
  arc A847 (-153.5, 161.675) -> (-150.325, 158.5) centre (-150.325, 161.675) ccw
  line L1275 (-153.5, 177.5) -> (-134.5, 158.5) construction
  arc A848 (-113.675, 158.5) -> (-110.5, 161.675) centre (-113.675, 161.675) ccw
  line L1276 (-129.5, 161.675) -> (-129.5, 174.325)
  line L1277 (-110.5, 174.325) -> (-110.5, 161.675)
  line L1278 (-110.5, 177.5) -> (-129.5, 158.5) construction
  arc A849 (-126.325, 177.5) -> (-129.5, 174.325) centre (-126.325, 174.325) ccw
  arc A850 (-110.5, 174.325) -> (-113.675, 177.5) centre (-113.675, 174.325) ccw
  line L1279 (-113.675, 158.5) -> (-126.325, 158.5)
  line L1280 (-126.325, 177.5) -> (-113.675, 177.5)
  arc A851 (-129.5, 161.675) -> (-126.325, 158.5) centre (-126.325, 161.675) ccw
  line L1281 (-129.5, 177.5) -> (-110.5, 158.5) construction
  arc A852 (-89.675, 158.5) -> (-86.5, 161.675) centre (-89.675, 161.675) ccw
  line L1282 (-105.5, 161.675) -> (-105.5, 174.325)
  line L1283 (-86.5, 174.325) -> (-86.5, 161.675)
  line L1284 (-86.5, 177.5) -> (-105.5, 158.5) construction
  arc A853 (-102.325, 177.5) -> (-105.5, 174.325) centre (-102.325, 174.325) ccw
  arc A854 (-86.5, 174.325) -> (-89.675, 177.5) centre (-89.675, 174.325) ccw
  line L1285 (-89.675, 158.5) -> (-102.325, 158.5)
  line L1286 (-102.325, 177.5) -> (-89.675, 177.5)
  arc A855 (-105.5, 161.675) -> (-102.325, 158.5) centre (-102.325, 161.675) ccw
  line L1287 (-105.5, 177.5) -> (-86.5, 158.5) construction
  arc A856 (-65.675, 158.5) -> (-62.5, 161.675) centre (-65.675, 161.675) ccw
  line L1288 (-81.5, 161.675) -> (-81.5, 174.325)
  line L1289 (-62.5, 174.325) -> (-62.5, 161.675)
  line L1290 (-62.5, 177.5) -> (-81.5, 158.5) construction
  arc A857 (-78.325, 177.5) -> (-81.5, 174.325) centre (-78.325, 174.325) ccw
  arc A858 (-62.5, 174.325) -> (-65.675, 177.5) centre (-65.675, 174.325) ccw
  line L1291 (-65.675, 158.5) -> (-78.325, 158.5)
  line L1292 (-78.325, 177.5) -> (-65.675, 177.5)
  arc A859 (-81.5, 161.675) -> (-78.325, 158.5) centre (-78.325, 161.675) ccw
  line L1293 (-81.5, 177.5) -> (-62.5, 158.5) construction
  arc A860 (-41.675, 158.5) -> (-38.5, 161.675) centre (-41.675, 161.675) ccw
  line L1294 (-57.5, 161.675) -> (-57.5, 174.325)
  line L1295 (-38.5, 174.325) -> (-38.5, 161.675)
  line L1296 (-38.5, 177.5) -> (-57.5, 158.5) construction
  arc A861 (-54.325, 177.5) -> (-57.5, 174.325) centre (-54.325, 174.325) ccw
  arc A862 (-38.5, 174.325) -> (-41.675, 177.5) centre (-41.675, 174.325) ccw
  line L1297 (-41.675, 158.5) -> (-54.325, 158.5)
  line L1298 (-54.325, 177.5) -> (-41.675, 177.5)
  arc A863 (-57.5, 161.675) -> (-54.325, 158.5) centre (-54.325, 161.675) ccw
  line L1299 (-57.5, 177.5) -> (-38.5, 158.5) construction
  arc A864 (-17.675, 158.5) -> (-14.5, 161.675) centre (-17.675, 161.675) ccw
  line L1300 (-33.5, 161.675) -> (-33.5, 174.325)
  line L1301 (-14.5, 174.325) -> (-14.5, 161.675)
  line L1302 (-14.5, 177.5) -> (-33.5, 158.5) construction
  arc A865 (-30.325, 177.5) -> (-33.5, 174.325) centre (-30.325, 174.325) ccw
  arc A866 (-14.5, 174.325) -> (-17.675, 177.5) centre (-17.675, 174.325) ccw
  line L1303 (-17.675, 158.5) -> (-30.325, 158.5)
  line L1304 (-30.325, 177.5) -> (-17.675, 177.5)
  arc A867 (-33.5, 161.675) -> (-30.325, 158.5) centre (-30.325, 161.675) ccw
  line L1305 (-33.5, 177.5) -> (-14.5, 158.5) construction
  arc A868 (6.325, 158.5) -> (9.5, 161.675) centre (6.325, 161.675) ccw
  line L1306 (-9.5, 161.675) -> (-9.5, 174.325)
  line L1307 (9.5, 174.325) -> (9.5, 161.675)
  line L1308 (9.5, 177.5) -> (-9.5, 158.5) construction
  arc A869 (-6.325, 177.5) -> (-9.5, 174.325) centre (-6.325, 174.325) ccw
  arc A870 (9.5, 174.325) -> (6.325, 177.5) centre (6.325, 174.325) ccw
  line L1309 (6.325, 158.5) -> (-6.325, 158.5)
  line L1310 (-6.325, 177.5) -> (6.325, 177.5)
  arc A871 (-9.5, 161.675) -> (-6.325, 158.5) centre (-6.325, 161.675) ccw
  line L1311 (-9.5, 177.5) -> (9.5, 158.5) construction
  arc A872 (30.325, 158.5) -> (33.5, 161.675) centre (30.325, 161.675) ccw
  line L1312 (14.5, 161.675) -> (14.5, 174.325)
  line L1313 (33.5, 174.325) -> (33.5, 161.675)
  line L1314 (33.5, 177.5) -> (14.5, 158.5) construction
  arc A873 (17.675, 177.5) -> (14.5, 174.325) centre (17.675, 174.325) ccw
  arc A874 (33.5, 174.325) -> (30.325, 177.5) centre (30.325, 174.325) ccw
  line L1315 (30.325, 158.5) -> (17.675, 158.5)
  line L1316 (17.675, 177.5) -> (30.325, 177.5)
  arc A875 (14.5, 161.675) -> (17.675, 158.5) centre (17.675, 161.675) ccw
  line L1317 (14.5, 177.5) -> (33.5, 158.5) construction
  arc A876 (54.325, 158.5) -> (57.5, 161.675) centre (54.325, 161.675) ccw
  line L1318 (38.5, 161.675) -> (38.5, 174.325)
  line L1319 (57.5, 174.325) -> (57.5, 161.675)
  line L1320 (57.5, 177.5) -> (38.5, 158.5) construction
  arc A877 (41.675, 177.5) -> (38.5, 174.325) centre (41.675, 174.325) ccw
  arc A878 (57.5, 174.325) -> (54.325, 177.5) centre (54.325, 174.325) ccw
  line L1321 (54.325, 158.5) -> (41.675, 158.5)
  line L1322 (41.675, 177.5) -> (54.325, 177.5)
  arc A879 (38.5, 161.675) -> (41.675, 158.5) centre (41.675, 161.675) ccw
  line L1323 (38.5, 177.5) -> (57.5, 158.5) construction
  arc A880 (78.325, 158.5) -> (81.5, 161.675) centre (78.325, 161.675) ccw
  line L1324 (62.5, 161.675) -> (62.5, 174.325)
  line L1325 (81.5, 174.325) -> (81.5, 161.675)
  line L1326 (81.5, 177.5) -> (62.5, 158.5) construction
  arc A881 (65.675, 177.5) -> (62.5, 174.325) centre (65.675, 174.325) ccw
  arc A882 (81.5, 174.325) -> (78.325, 177.5) centre (78.325, 174.325) ccw
  line L1327 (78.325, 158.5) -> (65.675, 158.5)
  line L1328 (65.675, 177.5) -> (78.325, 177.5)
  arc A883 (62.5, 161.675) -> (65.675, 158.5) centre (65.675, 161.675) ccw
  line L1329 (62.5, 177.5) -> (81.5, 158.5) construction
  arc A884 (102.325, 158.5) -> (105.5, 161.675) centre (102.325, 161.675) ccw
  line L1330 (86.5, 161.675) -> (86.5, 174.325)
  line L1331 (105.5, 174.325) -> (105.5, 161.675)
  line L1332 (105.5, 177.5) -> (86.5, 158.5) construction
  arc A885 (89.675, 177.5) -> (86.5, 174.325) centre (89.675, 174.325) ccw
  arc A886 (105.5, 174.325) -> (102.325, 177.5) centre (102.325, 174.325) ccw
  line L1333 (102.325, 158.5) -> (89.675, 158.5)
  line L1334 (89.675, 177.5) -> (102.325, 177.5)
  arc A887 (86.5, 161.675) -> (89.675, 158.5) centre (89.675, 161.675) ccw
  line L1335 (86.5, 177.5) -> (105.5, 158.5) construction
  arc A888 (126.325, 158.5) -> (129.5, 161.675) centre (126.325, 161.675) ccw
  line L1336 (110.5, 161.675) -> (110.5, 174.325)
  line L1337 (129.5, 174.325) -> (129.5, 161.675)
  line L1338 (129.5, 177.5) -> (110.5, 158.5) construction
  arc A889 (113.675, 177.5) -> (110.5, 174.325) centre (113.675, 174.325) ccw
  arc A890 (129.5, 174.325) -> (126.325, 177.5) centre (126.325, 174.325) ccw
  line L1339 (126.325, 158.5) -> (113.675, 158.5)
  line L1340 (113.675, 177.5) -> (126.325, 177.5)
  arc A891 (110.5, 161.675) -> (113.675, 158.5) centre (113.675, 161.675) ccw
  line L1341 (110.5, 177.5) -> (129.5, 158.5) construction
  arc A892 (150.325, 158.5) -> (153.5, 161.675) centre (150.325, 161.675) ccw
  line L1342 (134.5, 161.675) -> (134.5, 174.325)
  line L1343 (153.5, 174.325) -> (153.5, 161.675)
  line L1344 (153.5, 177.5) -> (134.5, 158.5) construction
  arc A893 (137.675, 177.5) -> (134.5, 174.325) centre (137.675, 174.325) ccw
  arc A894 (153.5, 174.325) -> (150.325, 177.5) centre (150.325, 174.325) ccw
  line L1345 (150.325, 158.5) -> (137.675, 158.5)
  line L1346 (137.675, 177.5) -> (150.325, 177.5)
  arc A895 (134.5, 161.675) -> (137.675, 158.5) centre (137.675, 161.675) ccw
  line L1347 (134.5, 177.5) -> (153.5, 158.5) construction
  arc A896 (174.325, 158.5) -> (177.5, 161.675) centre (174.325, 161.675) ccw
  line L1348 (158.5, 161.675) -> (158.5, 174.325)
  line L1349 (177.5, 174.325) -> (177.5, 161.675)
  line L1350 (177.5, 177.5) -> (158.5, 158.5) construction
  arc A897 (161.675, 177.5) -> (158.5, 174.325) centre (161.675, 174.325) ccw
  arc A898 (177.5, 174.325) -> (174.325, 177.5) centre (174.325, 174.325) ccw
  line L1351 (174.325, 158.5) -> (161.675, 158.5)
  line L1352 (161.675, 177.5) -> (174.325, 177.5)
  arc A899 (158.5, 161.675) -> (161.675, 158.5) centre (161.675, 161.675) ccw
  line L1353 (158.5, 177.5) -> (177.5, 158.5) construction
  dimension "d5" = 19
  dimension "d6" = 19
  dimension "d7" = 3.175
  dimension "d8" = 3.175
  dimension "d9" = 3.175
  dimension "d10" = 3.175
  dimension "d13" = 24
  dimension "d14" = 24
  constraint perpendicular L4 L5
  constraint parallel L4 L6
  constraint parallel L5 L7
  constraint horizontal L4
  constraint coincident L8 origin
  constraint coincident L9 origin
  constraint coincident L6
  constraint coincident L5
  constraint tangent L6 A0
  constraint tangent L5 A0
  constraint coincident L7
  constraint tangent L6 A1
  constraint tangent L7 A1
  constraint coincident L4
  constraint tangent L4 A2
  constraint tangent L7 A2
  constraint tangent L4 A3
  constraint tangent L5 A3
  measures "d7" radius of A0
  measures "d8" radius of A1
  measures "d9" radius of A2
  measures "d10" radius of A3